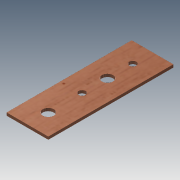
# Autodesk Inventor part: gabatarito-rolamento
Saved by Autodesk Inventor 2017 (Build 210142000, 142)
## iProperties
Created: 2018-08-18
Part Number: gabatarito-rolamento
Material: Wood (Oak)
Document SubType Name: Sheet Metal
Designer: Luiz Gustavo
Density: 0.76 g/cm^3
Sheet Metal Rule: Default_mm
Appearance: White Oak - Natural Medium Gloss
Author: Luiz Gustavo
Autodesk Inventor part; units mm, degrees
ref_plane "YZ Plane" through (0, 0, 0) normal (1, 0, 0) x (0, 1, 0)
ref_plane "XZ Plane" through (0, 0, 0) normal (0, 1, 0) x (-1, 0, 0)
ref_plane "XY Plane" through (0, 0, 0) normal (0, 0, 1) x (1, 0, 0)
sketch "Sketch1" plane through (0, 0, 0) normal (0, 0, 1) x (1, 0, 0)
  ellipse E0 centre (-4.5001, 27.5565) end of major axis (-7.5001, 27.5565) minor radius 3
  line L0 (-2.0001, 9.3017) -> (-2.0001, 9.2846)
  line L1 (-2.0001, 45.8017) -> (-2.0001, 45.7846)
  line L2 (-1445.7599, 60) -> (10.4999, 60)
  line L3 (-19.4999, -29.9999) -> (-19.4999, 60)
  line L4 (10.4999, -29.9999) -> (10.4999, 60)
  line L5 (8.4999, -29.9999) -> (0, -29.9999)
  line L6 (10.4999, -29.9999) -> (-19.4999, -29.9999)
  line L7 (-19.4999, -29.9999) -> (-19.4999, 60)
  line L8 (-19.4999, 60) -> (10.4999, 60)
  line L9 (10.4999, 60) -> (10.4999, -29.9999)
  circle A0 centre (-4.5001, 27.5565) radius 4
  circle A1 centre (-4.5001, 45.8024) radius 2.5
  circle A2 centre (-4.5001, 9.3024) radius 2.5
  line L10 (-4.5, -29.9999) -> (-4.5, -14.9999) construction
  circle A3 centre (-4.5, -14.9999) radius 4
  point P0 (0, 0)
  dimension "d0" = 8
  dimension "d1" = 5
  dimension "d2" = 89.9999
  dimension "d3" = 15
  dimension "d4" = 8
  measures "d0" diameter of A0
  measures "d1" diameter of A1
  measures "d2" distance of L4.start L4.end
  measures "d3" distance of L10.start L10.end
  measures "d4" diameter of A3
extrude "Plate1" add sketch "Sketch1" along normal blind 2 contours L2 L4 L6 L5 L3
equation "\"BendRadius\" = Thickness"
equation "\"BendReliefWidth\" = Thickness"
equation "\"BendReliefDepth\" = 0.5 * Thickness"
equation "\"CornerReliefSize\" = 4 * Thickness"
equation "\"MinimumRemnant\" = 2 * Thickness"
equation "\"TransitionRadius\" = BendRadius"
equation "\"JacobiRadiusSize\" = BendRadius"
equation "\"GapSize\" = Thickness"
equation "\"d5\" = BendRadius"
equation "\"Thickness\" = 2"
body "Solid1"
